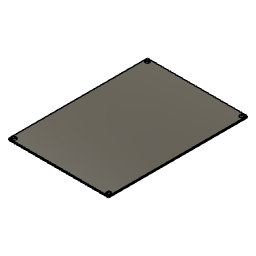
substrate1 (Autodesk Fusion 360 design; units mm, degrees)
Autodesk Fusion 360 part; units mm, degrees
sketch "スケッチ1" plane through (0, 0, 0) normal (0, 0, 1) x (1, 0, 0)
  line L0 (0, 0) -> (68.58, 0)
  line L1 (0, 0) -> (68.58, 0)
  line L2 (68.58, 0) -> (68.58, 96.52)
  line L3 (68.58, 96.52) -> (0, 96.52)
  line L4 (0, 96.52) -> (0, 0)
  circle A0 centre (0, 0) radius 1.5
  circle A1 centre (68.58, 0) radius 1.5
  circle A2 centre (0, 96.52) radius 1.5
  circle A3 centre (68.58, 96.52) radius 1.5
  line L5 (-5, -5) -> (73.58, -5)
  line L6 (73.58, -5) -> (73.58, 101.52)
  line L7 (73.58, 101.52) -> (-5, 101.52)
  line L8 (-5, 101.52) -> (-5, -5)
  dimension "d1" = 68.58
  dimension "d2" = 68.58
  dimension "d3" = 96.52
  dimension "d4" = 3
  dimension "d5" = 3
  dimension "d6" = 3
  dimension "d7" = 3
  dimension "d8" = 78.58
  dimension "d9" = 106.52
  constraint coincident L0.start L1.start
  constraint horizontal L0
  constraint horizontal L1
  constraint vertical L2
  constraint horizontal L3
  constraint vertical L4
  constraint coincident L0.end L1.end
  constraint coincident L3.end L4.start
  constraint coincident L2.end L3.start
  constraint horizontal L5
  constraint vertical L6
  constraint horizontal L7
  constraint vertical L8
  measures "d1" distance of L0.start L0.end
  measures "d2" distance of L0.start L0.end
  measures "d3" distance of L0.start L3.end
  measures "d4" diameter of A0
  measures "d5" diameter of A1
  measures "d6" diameter of A2
  measures "d7" diameter of A3
  measures "d8" distance of L5.start L5.end
  measures "d9" distance of L5.start L7.end
extrude "押し出し1" add sketch "スケッチ1" along normal blind 2 contours L0 L1 L2 L3 L4 A0 A1 A2 A3 | L5 L6 L7 L8
sketch "スケッチ2" plane through (0, 0, 2) normal (0, 0, 1) x (-1, 0, 0)
  circle A0 centre (0, 0) radius 1.5
  circle A1 centre (-68.58, -96.52) radius 1.5
  circle A2 centre (0, -96.52) radius 1.5
  circle A3 centre (-68.58, 0) radius 1.5
  line L0 (5, -101.52) -> (5, 5)
  line L1 (5, 5) -> (-73.58, 5)
  line L2 (-73.58, 5) -> (-73.58, -101.52)
  line L3 (-73.58, -101.52) -> (5, -101.52)
  line L4 (5, 2.0966) -> (-73.58, 2.0966)
  line L5 (1.9893, 5) -> (1.9893, -101.52)
  line L6 (-70.5693, 5) -> (-70.5693, -101.52)
  line L7 (5, -98.6166) -> (-73.58, -98.6166)
  constraint coincident L0 L4.start
  constraint coincident L2 L4.end
  constraint perpendicular L2 L4
  constraint coincident L1 L5.start
  constraint coincident L3 L5.end
  constraint perpendicular L3 L5
extrude "押し出し2" cut sketch "スケッチ2" against normal blind 2 contours L0 L3 L5 L7 | L0 L4 L5 L7 | L3 L5 L6 L7 | L0 L1 L4 L5 | L2 L3 L6 L7 | L1 L4 L5 L6 | L2 L4 L6 L7 | L1 L2 L4 L6
extrude "押し出し3" cut 1 faces at (45.4465, 32.5919, 2) along direction (0, 0, -1) blind 1
